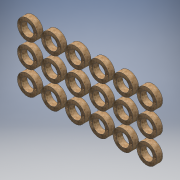
# Autodesk Inventor part: BearingSiliconeMoldSpacer
Saved by Autodesk Inventor 2016 (Build 200138000, 138)
## iProperties
Created: 2015-12-06
Part Number: BearingSiliconeMoldSpacer
Material: MDF Medium Density Fiberboard
Document SubType Name: Modeling
Designer: DonMo
Density: 0.8 g/cm^3
Appearance: Cardboard - Corrugated
Author: DonMo
Autodesk Inventor part; units mm, degrees
ref_plane "YZ Plane" through (0, 0, 0) normal (1, 0, 0) x (0, 1, 0)
ref_plane "XZ Plane" through (0, 0, 0) normal (0, 1, 0) x (-1, 0, 0)
ref_plane "XY Plane" through (0, 0, 0) normal (0, 0, 1) x (1, 0, 0)
sketch "Sketch1" plane through (0, 0, 0) normal (0, 1, 0) x (-1, 0, 0)
  circle A0 centre (0, 0) radius 7 construction
  circle A1 centre (0, 0) radius 3.175
  line L0 (7, -31) -> (-67, -31) construction
  line L1 (-67, -31) -> (-67, 7) construction
  line L2 (-67, 7) -> (7, 7) construction
  line L3 (7, 7) -> (7, -31) construction
  circle A2 centre (0, 0) radius 5
  line L4 (0, 0) -> (-3.175, 0) construction
  line L5 (0, 0) -> (0, -3.175) construction
  circle A3 centre (-12, 0) radius 5
  circle A4 centre (-12, 0) radius 3.175
  circle A5 centre (-24, 0) radius 5
  circle A6 centre (-24, 0) radius 3.175
  circle A7 centre (-36, 0) radius 5
  circle A8 centre (-36, 0) radius 3.175
  circle A9 centre (-48, 0) radius 5
  circle A10 centre (-48, 0) radius 3.175
  circle A11 centre (-60, 0) radius 5
  circle A12 centre (-60, 0) radius 3.175
  circle A13 centre (0, -12) radius 5
  circle A14 centre (0, -12) radius 3.175
  circle A15 centre (-12, -12) radius 5
  circle A16 centre (-12, -12) radius 3.175
  circle A17 centre (-24, -12) radius 5
  circle A18 centre (-24, -12) radius 3.175
  circle A19 centre (-36, -12) radius 5
  circle A20 centre (-36, -12) radius 3.175
  circle A21 centre (-48, -12) radius 5
  circle A22 centre (-48, -12) radius 3.175
  circle A23 centre (-60, -12) radius 5
  circle A24 centre (-60, -12) radius 3.175
  circle A25 centre (0, -24) radius 5
  circle A26 centre (0, -24) radius 3.175
  circle A27 centre (-12, -24) radius 5
  circle A28 centre (-12, -24) radius 3.175
  circle A29 centre (-24, -24) radius 5
  circle A30 centre (-24, -24) radius 3.175
  circle A31 centre (-36, -24) radius 5
  circle A32 centre (-36, -24) radius 3.175
  circle A33 centre (-48, -24) radius 5
  circle A34 centre (-48, -24) radius 3.175
  circle A35 centre (-60, -24) radius 5
  circle A36 centre (-60, -24) radius 3.175
  point P0 (-15.175, 0)
  point P1 (-12, -3.175)
  point P2 (-27.175, 0)
  point P3 (-24, -3.175)
  point P4 (-39.175, 0)
  point P5 (-36, -3.175)
  point P6 (-51.175, 0)
  point P7 (-48, -3.175)
  point P8 (-63.175, 0)
  point P9 (-60, -3.175)
  point P10 (-3.175, -12)
  point P11 (0, -15.175)
  point P12 (-15.175, -12)
  point P13 (-12, -15.175)
  point P14 (-27.175, -12)
  point P15 (-24, -15.175)
  point P16 (-39.175, -12)
  point P17 (-36, -15.175)
  point P18 (-51.175, -12)
  point P19 (-48, -15.175)
  point P20 (-63.175, -12)
  point P21 (-60, -15.175)
  point P22 (-3.175, -24)
  point P23 (0, -27.175)
  point P24 (-15.175, -24)
  point P25 (-12, -27.175)
  point P26 (-27.175, -24)
  point P27 (-24, -27.175)
  point P28 (-39.175, -24)
  point P29 (-36, -27.175)
  point P30 (-51.175, -24)
  point P31 (-48, -27.175)
  point P32 (-63.175, -24)
  point P33 (-60, -27.175)
  dimension "d6" = 6.35
  dimension "d21" = 14
  dimension "d22" = 10
  dimension "d25" = 12
  dimension "d28" = 12
  dimension "d32" = 2
  dimension "d33" = 2
  dimension "d34" = 74
  dimension "d35" = 38
  constraints: 37 centre point, 36 point on circle, 19 coincident, 12 end point, 3 horizontal, 2 parallel, 2 perpendicular, 2 tangent, 1 concentric, 1 vertical, 102 other
  measures "d6" diameter of A1
  measures "d21" diameter of A0
  measures "d22" diameter of A2
  measures "d25" distance of L4.start A3.centre
  measures "d28" distance of L4.start A13.centre
  measures "d32" distance edge to line of A29 L0
  measures "d33" distance edge to line of A11 L1
  measures "d34" distance of L1.end L2.end
  measures "d35" distance of L0.end L1.end
extrude "Extrusion2" add sketch "Sketch1" along normal blind 3
equation "\"d6\" = DowlDiameter"
equation "\"BearingDiameter\" = 24"
equation "\"DowlDiameter\" = 6.35"
body "Solid2"
